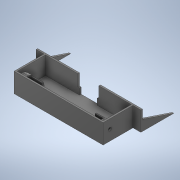
# Autodesk Inventor part: BodyV2
Saved by Autodesk Inventor 2020 (Build 240168000, 168)
## iProperties
Created: 2023-11-26
Part Number: BodyV2
Material: Thermoplastic Resin
Document SubType Name: Modeling
Designer: smz3rm
Density: 1.28 g/cm^3
Appearance: Smooth - Black
Mass: 125.446 g
Surface Area: 571.471 cm^2
Volume: 98.0049 cm^3
Author: smz3rm
Autodesk Inventor part; units mm, degrees
ref_plane "YZ Plane" through (0, 0, 0) normal (1, 0, 0) x (0, 1, 0)
ref_plane "XZ Plane" through (0, 0, 0) normal (0, 1, 0) x (-1, 0, 0)
ref_plane "XY Plane" through (0, 0, 0) normal (0, 0, 1) x (1, 0, 0)
sketch "Sketch1" plane through (0, 0, 0) normal (0, 1, 0) x (-1, 0, 0)
  line L0 (85, 30) -> (-85, 30)
  line L1 (-85, 30) -> (-85, -30)
  line L2 (-85, -30) -> (85, -30)
  line L3 (85, -30) -> (85, 30)
  line L4 (85, 30) -> (-85, -30) construction
  line L5 (-85, 30) -> (85, -30) construction
  line L6 (-85, -30) -> (-100, -30)
  line L7 (-100, -30) -> (-100, -27)
  line L8 (-100, -27) -> (-85, -27)
  line L9 (0, -42) -> (0, 42) projected
  line L10 (85, -30) -> (100, -30)
  line L11 (100, -30) -> (100, -27)
  line L12 (100, -27) -> (85, -27)
  point P0 (0, 0)
  point P1 (85, -27)
  dimension "d0" = 170
  dimension "d1" = 60
  dimension "d32" = 15
  dimension "d33" = 3
  constraints: 24 end point, 3 symmetric about line, 2 midpoint, 2 parallel, 2 perpendicular, 2 point on line, 1 horizontal, 1 vertical
  measures "d0" distance of L2.end L1.end
  measures "d1" distance of L1.end L0.end
  measures "d32" distance of L1.end L6.end
  measures "d33" distance of L6.end L7.end
extrude "Extrusion1" add sketch "Sketch1" along normal blind 3
sketch "Sketch2" plane through (0, 3, 0) normal (0, 1, 0) x (1, 0, 0)
  line L0 (-85, 27) -> (-85, -30) projected
  line L1 (-85, -30) -> (85, -30) projected
  line L2 (85, -30) -> (85, 27) projected
  line L3 (100, 30) -> (-100, 30) projected
  line L4 (-100, 30) -> (-100, 27) projected
  line L5 (-100, 27) -> (-85, 27) projected
  line L6 (85, 27) -> (100, 27) projected
  line L7 (100, 27) -> (100, 30) projected
  line L8 (82, -27) -> (-82, -27)
  line L9 (-82, -27) -> (-82, 27)
  line L10 (-82, 27) -> (82, 27)
  line L11 (82, 27) -> (82, -27)
  line L12 (82, -27) -> (-82, 27) construction
  line L13 (-82, -27) -> (82, 27) construction
  point P0 (0, 0)
  dimension "d36" = 164
  dimension "d37" = 54
  constraints: 12 end point, 2 midpoint, 2 parallel, 1 horizontal, 1 perpendicular
  measures "d36" distance of L9.end L10.end
  measures "d37" distance between parallel lines of L10 L8
extrude "Extrusion2" add sketch "Sketch2" along normal blind 34
sketch "Sketch7" plane through (-82, 3, 27) normal (1, 0, 0) x (0, 0, -1)
  circle A0 centre (10, 17) radius 8
  line L0 (54, -3) -> (-3, -3) projected
  circle A1 centre (10, 17) radius 10
  line L1 (0, 17) -> (0, 0)
  line L2 (0, 17) -> (20, 17)
  line L3 (20, 17) -> (20, 0)
  line L4 (-3, -3) -> (-3, 34) projected
  line L5 (0, 0) -> (20, 0)
  line L6 (10, 27) -> (0, 27)
  line L7 (0, 0) -> (0, 34) projected
  line L8 (0, 17) -> (0, 27)
  point P0 (27, -3)
  point P1 (57, -3)
  dimension "d17" = 16
  dimension "d18" = 20
  dimension "d20" = 2
  dimension "d40" = 20
  dimension "d62" = 10
  constraints: 12 end point, 3 horizontal, 3 point on circle, 2 centre point, 2 vertical, 1 perpendicular, 1 point on line
  measures "d17" diameter of A0
  measures "d18" distance from line of L0 A0.centre
  measures "d20" radial gap between concentric circles of A0 A1
  measures "d40" distance between parallel lines of L3 L1
  measures "d62" distance of L6.start L6.end
extrude "Extrusion5" add sketch "Sketch7" along normal blind 11.25 contours L2 A1 A0 | A0 L2 A1 | L3 L5 L1 A1 | L7 L6 A1
sketch "Sketch8" plane through (-70.75, 3, 27) normal (1, 0, 0) x (0, 0, -1)
  arc A0 (20, 17) -> (10, 27) centre (10, 17) ccw projected
  circle A1 centre (10, 17) radius 8 projected
  line L0 (0, 0) -> (0, 27) projected
  line L1 (20, 0) -> (0, 0) projected
  line L2 (20, 0) -> (20, 17) projected
  circle A2 centre (10, 17) radius 7.75
  line L3 (10, 27) -> (0, 27) projected
  line L4 (0, 0) -> (0, 27) projected
  line L5 (4, 12.0946) -> (4, 22.2915)
  line L6 (10, 27) -> (0, 27) projected
  line L7 (16, 12.0946) -> (16, 22.2915)
  line L8 (16, 22.2915) -> (18.4853, 22.2915)
  arc A3 (20, 17) -> (10, 27) centre (10, 17) ccw projected
  line L9 (4, 22.2915) -> (0, 22.2915)
  point P0 (27, -3)
  point P1 (4, 27)
  point P2 (18.4853, 22.2915)
  point P3 (4, 21.9054)
  point P4 (16, 21.9054)
  dimension "d55" = 15.5
  dimension "d63" = 12
  dimension "d64" = 6
  constraints: 8 end point, 6 point on circle, 2 perpendicular, 2 point on line, 1 centre point, 1 coincident, 1 horizontal, 1 vertical
  measures "d55" diameter of A2
  measures "d63" distance between parallel lines of L7 L5
  measures "d64" distance from line of L5 point (10, 17)
extrude "Extrusion6" add sketch "Sketch8" along normal blind 20 contours L2 L1 L0 L9 A1 L8 A0 | A1 L5 A2 L7 | A2 L7 | L5 A2 picked at (9.114, 9.2488)
sketch "Sketch9" plane through (-82, 20, 17) normal (1, 0, 0) x (0, 0, -1)
  circle A0 centre (0, 0) radius 3
  line L0 (44, -20) -> (-13, -20) projected
  line L1 (-13, -20) -> (-13, 17) projected
  point P0 (17, -20)
  point P1 (47, -20)
  dimension "d27" = 6
  dimension "d28" = 20
  dimension "d41" = 13
  constraints: 1 centre point
  measures "d27" diameter of A0
  measures "d28" distance from line of L0 A0.centre
  measures "d41" distance from line of L1 A0.centre
extrude "Extrusion7" cut sketch "Sketch9" against normal up to surface (3 mm away)
mirror "Mirror2" about plane through (0, 0, 0) normal (1, 0, 0) of "Extrusion7", "Extrusion6", "Extrusion5"
sketch "Sketch4" plane through (-87, 3, -27) normal (0, 0, 1) x (1, 0, 0)
  line L0 (87, 34) -> (107, 34)
  line L1 (87, 34) -> (67, 34)
  line L2 (67, 34) -> (67, 0)
  line L3 (107, 34) -> (107, 0)
  line L4 (107, 0) -> (67, 0)
  line L5 (5, 0) -> (5, 34) projected
  line L6 (5, 34) -> (169, 34) projected
  line L7 (67, 12) -> (70, 12)
  line L8 (70, 12) -> (70, 0)
  line L9 (107, 12) -> (104, 12)
  line L10 (104, 12) -> (104, 0)
  point P0 (87, -3)
  dimension "d13" = 20
  dimension "d14" = 20
  dimension "d42" = 82
  dimension "d43" = 34
  dimension "WeaponMountThickness" = 3
  dimension "WeaponMountSlot" = 12
  constraints: 18 end point, 4 horizontal, 4 perpendicular, 4 point on line, 2 equal length, 1 collinear, 1 vertical
  measures "d13" distance of L0.start L0.end
  measures "d14" distance of L0.start L1.end
  measures "d42" distance from line of L5 L0.start
  measures "d43" distance of L1.end L2.end
  measures "WeaponMountThickness" distance of L7.start L7.end
  measures "WeaponMountSlot" distance of L7.end L8.end
extrude "Extrusion9" cut sketch "Sketch4" against normal up to surface (3 mm away) contours L0 L3 L9 L10 L4 L8 L7 L2 L1
sketch "Sketch13" plane through (100, 0, -27) normal (1, 0, 0) x (0, 0, -1)
  line L0 (0, 0) -> (3, 0) projected
  line L1 (3, 0) -> (3, 20)
  line L2 (0, 0) -> (0, 37) projected
  line L3 (3, 20) -> (63, 0)
  line L4 (63, 0) -> (3, 0)
  point P0 (-27, 0)
  dimension "d60" = 60
  dimension "d61" = 20
  constraints: 6 end point, 1 parallel, 1 perpendicular
  measures "d60" distance of L3.end L0.end
  measures "d61" distance of L0.end L1.end
extrude "Extrusion11" add sketch "Sketch13" against normal blind 3
mirror "Mirror4" about plane through (0, 0, 0) normal (1, 0, 0) of "Extrusion11"
sketch "Sketch14" plane through (0, 3, 0) normal (0, 1, 0) x (1, 0, 0)
  point P0 (0, 0)
equation "\"d0\" = Width"
equation "\"d1\" = Length"
equation "\"d32\" = -0.5 * Width + 0.5 * FullWidth"
equation "\"d33\" = SideWallThickness"
equation "\"d2\" = BaseWallThickness"
equation "\"d36\" = Width - 2 * SideWallThickness"
equation "\"d37\" = Length - 2 * SideWallThickness"
equation "\"d5\" = Height - 2 * BaseWallThickness"
equation "\"d18\" = DriveMotorHeight"
equation "\"d20\" = DriveMotorMountThickness"
equation "\"d28\" = DriveMotorHeight"
equation "\"d13\" = 0.5 * WeaponSlotWidth"
equation "\"d14\" = 0.5 * WeaponSlotWidth"
equation "\"d42\" = 0.5 * Width - SideWallThickness"
equation "\"d43\" = Height - 2 * BaseWallThickness"
equation "\"d60\" = WedgeLength"
equation "\"d61\" = WedgeHeight"
equation "\"d53\" = SideWallThickness"
equation "\"SideWallThickness\" = 3"
equation "\"BaseWallThickness\" = 3"
equation "\"Width\" = 170"
equation "\"Length\" = 60"
equation "\"DriveMotorHeight\" = 20"
equation "\"DriveMotorMountThickness\" = 2"
equation "\"WedgeLength\" = 60"
equation "\"WedgeHeight\" = 20"
equation "\"FullWidth\" = 200"
equation "\"Height\" = 40"
equation "\"WeaponSlotWidth\" = 40"
body "Solid1"
